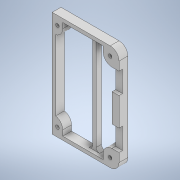
# Autodesk Inventor part: atx-adapter_cable-press
Saved by Autodesk Inventor 2021 (Build 250183000, 183)
## iProperties
Created: 2024-03-19
Part Number: atx-adapter_cable-press
Material: Generic
Document SubType Name: Modeling
Designer: Toby
Density: 1 g/cm^3
Appearance: Default
Author: Toby
Autodesk Inventor part; units mm, degrees
ref_plane "YZ Plane" through (0, 0, 0) normal (1, 0, 0) x (0, 1, 0)
ref_plane "XZ Plane" through (0, 0, 0) normal (0, 1, 0) x (-1, 0, 0)
ref_plane "XY Plane" through (0, 0, 0) normal (0, 0, 1) x (1, 0, 0)
sketch "Sketch1" plane through (0, 0, 0) normal (0, 0, 1) x (1, 0, 0)
  line L0 (-34.9037, 22.6593) -> (3.0963, 22.6593)
  line L1 (3.0963, 22.6593) -> (3.0963, -37.3407)
  line L2 (3.0963, -37.3407) -> (-34.9037, -37.3407)
  line L3 (-34.9037, -37.3407) -> (-34.9037, 22.6593)
  point P0 (0, 0)
  dimension "d0" = 38
  dimension "d1" = 60
  constraints: 8 end point, 2 parallel, 1 horizontal, 1 perpendicular
  measures "d0" distance of L0.start L0.end
  measures "d1" distance of L2.end L0.start
extrude "Extrusion1" add sketch "Sketch1" along normal blind 5
sketch "Sketch2" plane through (0, 0, 5) normal (0, 0, 1) x (1, 0, 0)
  line L0 (3.0963, -37.3407) -> (3.0963, 22.6593) projected
  line L1 (3.0963, 22.6593) -> (-34.9037, 22.6593) projected
  line L2 (-34.9037, -37.3407) -> (3.0963, -37.3407) projected
  point P0 (0, 0)
  point P1 (-31.9037, 17.6593)
  point P2 (-1.9037, 17.6593)
  point P3 (-31.9037, -32.3407)
  point P4 (-1.9037, -32.3407)
  dimension "d4" = 30
  dimension "d5" = 30
  dimension "d6" = 5
  dimension "d7" = 5
  dimension "d8" = 5
  dimension "d9" = 5
  dimension "d10" = 5
  dimension "d11" = 5
  measures "d4" distance of point (-1.904, 17.659) point (-31.904, 17.659)
  measures "d5" distance of point (-31.904, -32.341) point (-1.904, -32.341)
  measures "d6" distance from line of L0 point (-1.904, 17.659)
  measures "d7" distance from line of L1 point (-1.904, 17.659)
  measures "d8" distance from line of L1 point (-31.904, 17.659)
  measures "d9" distance from line of L0 point (-1.904, -32.341)
  measures "d10" distance from line of L2 point (-1.904, -32.341)
  measures "d11" distance from line of L2 point (-31.904, -32.341)
hole "Hole1" at (-31.9037, 17.6593, 5) at (-1.9037, 17.6593, 5) at (-31.9037, -32.3407, 5) at (-1.9037, -32.3407, 5) direction (0, 0, -1) diameter 2 depth 10 tip angle 118
sketch "Sketch3" plane through (0, 0, 5) normal (0, 0, 1) x (1, 0, 0)
  line L0 (-28.9037, 20.6593) -> (-5.9037, 20.6593)
  line L1 (-5.9037, 20.6593) -> (-5.9037, -35.3407)
  line L2 (-5.9037, -35.3407) -> (-28.9037, -35.3407)
  line L3 (-28.9037, -35.3407) -> (-28.9037, 20.6593)
  line L4 (-32.9037, 12.6593) -> (-0.795, 12.6593)
  line L5 (-0.795, 12.6593) -> (-0.795, -27.3407)
  line L6 (-0.795, -27.3407) -> (-32.9037, -27.3407)
  line L7 (-32.9037, -27.3407) -> (-32.9037, 12.6593)
  line L8 (-34.9037, 22.6593) -> (-34.9037, -37.3407) projected
  line L9 (3.0963, -37.3407) -> (3.0963, 22.6593) projected
  line L10 (3.0963, 22.6593) -> (-34.9037, 22.6593) projected
  line L11 (-34.9037, -37.3407) -> (3.0963, -37.3407) projected
  point P0 (0, 0)
  point P1 (-28.9037, 12.6593)
  point P2 (-28.9037, -27.3407)
  point P3 (-5.9037, -27.3407)
  point P4 (-5.9037, 12.6593)
  dimension "d19" = 2
  dimension "d20" = 3.8913
  dimension "d21" = 2
  dimension "d22" = 2
  dimension "d23" = 6
  dimension "d24" = 9
  dimension "d25" = 10
  dimension "d26" = 10
  constraints: 16 end point, 4 parallel, 2 horizontal, 2 perpendicular
  measures "d19" distance between parallel lines of L8 L7
  measures "d20" distance between parallel lines of L9 L5
  measures "d21" distance between parallel lines of L0 L10
  measures "d22" distance between parallel lines of L11 L2
  measures "d23" distance between parallel lines of L8 L3
  measures "d24" distance between parallel lines of L9 L1
  measures "d25" distance between parallel lines of L10 L4
  measures "d26" distance between parallel lines of L11 L6
extrude "Extrusion2" cut sketch "Sketch3" against normal blind 5 contours L0 L1 L4 L3 | L4 L1 L6 L3 | L3 L6 L7 L4 | L4 L5 L6 L1 | L6 L1 L2 L3
sketch "Sketch4" plane through (3.0963, -37.3407, 0) normal (1, 0, 0) x (0, 0, -1)
  line L0 (-5, 50) -> (-3, 50)
  line L1 (-3, 50) -> (-3, 38)
  line L2 (-3, 38) -> (-5, 38)
  line L3 (-5, 38) -> (-5, 50)
  line L4 (-5, 60) -> (-5, 0) projected
  line L5 (-5, 10) -> (-3, 10)
  line L6 (-3, 10) -> (-3, 22)
  line L7 (-3, 22) -> (-5, 22)
  line L8 (-5, 22) -> (-5, 10)
  line L9 (-5, 10) -> (0, 10) projected
  line L10 (-5, 50) -> (0, 50) projected
  point P0 (0, 37.3407)
  dimension "d29" = 12
  dimension "d30" = 12
  dimension "d31" = 0
  dimension "d32" = 2
  constraints: 16 end point, 4 parallel, 2 collinear, 2 horizontal, 2 perpendicular, 2 point on line
  measures "d29" distance of L0.end L1.end
  measures "d30" distance of L5.end L6.end
  measures "d31" distance between parallel lines of L9 L5
  measures "d32" distance between parallel lines of L3 L1
extrude "Extrusion3" cut sketch "Sketch4" against normal blind 5
fillet "Fillet1" radius 5 2 edges at (3.0963, 22.6593, 2.5) (3.0963, -37.3407, 2.5)
sketch "Sketch5" plane through (0, 0, 0) normal (0, 0, -1) x (-1, 0, 0)
  line L0 (5.9037, 20.6593) -> (28.9037, 20.6593) projected
  line L1 (13.9037, 20.6593) -> (11.9037, 20.6593)
  line L2 (11.9037, 20.6593) -> (11.9037, -35.3407)
  line L3 (11.9037, -35.3407) -> (13.9037, -35.3407)
  line L4 (13.9037, -35.3407) -> (13.9037, 20.6593)
  line L5 (-3.0963, -32.3407) -> (-3.0963, 17.6593) projected
  line L6 (28.9037, -35.3407) -> (5.9037, -35.3407) projected
  point P0 (0, 0)
  dimension "d36" = 15
  dimension "d37" = 2
  constraints: 8 end point, 2 parallel, 1 collinear, 1 horizontal, 1 perpendicular, 1 point on line
  measures "d36" distance between parallel lines of L5 L2
  measures "d37" distance between parallel lines of L2 L4
extrude "Extrusion4" add sketch "Sketch5" against normal blind 3
fillet "Fillet2" radius 5 4 edges at (-28.9037, 12.6593, 2.5) (-28.9037, -27.3407, 2.5) (-5.9037, -27.3407, 2.5) (-5.9037, 12.6593, 2.5)
fillet "Fillet3" radius 2 4 edges at (-13.9037, 20.6593, 1.5) (-11.9037, 20.6593, 1.5) (-11.9037, -35.3407, 1.5) (-13.9037, -35.3407, 1.5)
body "Solid1"
